Ball system_v13 (Autodesk Fusion 360 design; units mm, degrees)
Autodesk Fusion 360 part; units mm, degrees
sketch "Esquisse3" plane through (0, 0, 0) normal (1, 0, 0) x (0, 1, 0) in component "Ball unit"
  line L0 (0, 26) -> (0, 30)
  circle A0 centre (0, 20) radius 10
  line L1 (0, 0) -> (0, 20) construction
  line L2 (0, 0) -> (0, 10) construction
  line L3 (0, 20) -> (10, 20) construction
  line L4 (10, 20) -> (-10, 20)
  dimension "d8" = 4
  dimension "d9" = 20
  dimension "d10" = 20
  constraint vertical L0
  constraint coincident L0.end A0
  constraint coincident L1.start L2.start
  constraint coincident A0.centre L1.end
  constraint vertical L1
  constraint midpoint L1 L2.end
  constraint coincident A0 L3.end
  constraint perpendicular L1 L3
  constraint coincident A0 L4.end
  constraint perpendicular L1 L4
  measures "d8" distance of L0.start L0.end
  measures "d9" diameter of A0
  measures "d10" distance of L1.start A0.centre
sketch "Esquisse1" plane through (0, 0, 0) normal (0, 0, 1) x (1, 0, 0) in component "Ball unit"
  circle A0 centre (0, 0) radius 15
  circle A1 centre (0, 0) radius 4
  dimension "d1" = 30
  dimension "d2" = 8
  constraint coincident A0.centre A1.centre
  constraint concentric A0 A1
  measures "d1" diameter of A0
  measures "d2" diameter of A1
extrude "Extrusion1" add sketch "Esquisse1" along normal blind 26 contours A0 | A1 makes body 1 in component "Ball unit"
extrude "Extrusion2" add sketch "Esquisse1" against normal blind 25 contours A1 bodies 1 in component "Ball unit"
thread "Filetage1" "ISO Metric profile 8.0 M8x1.25 6g" major diameter 7.866 minor diameter 6.4455 pitch 1.25 angle 60 resizes the face on face at (3.9801, -0.3983, -8.3333) on bodies 1 in component "Ball unit"
sketch "Esquisse2" plane through (0, 0, 26) normal (0, 0, 1) x (-1, 0, 0) in component "Ball unit"
  circle A0 centre (0, 0) radius 15
  circle A1 centre (0, 0) radius 8.25
  dimension "d7" = 16.5
  constraint coincident A0.centre A1.centre
  measures "d7" diameter of A1
revolve "Révolution1" add sketch "Esquisse3" angle 360 about axis through (0, 10, 20) along (0, -1, 0) contours A0 L4 picked at (-0.0339, 23.8077) bodies 1 in component "Ball unit"
fillet "Congé1" radius 1 1 edges at (-13.9849, -5.4242, 26) on bodies 1 in component "Ball unit"
copy_body "CutPasteBodies1" bodies 1 removing the originals makes body 2 in component "Ball unit"
sketch "Esquisse1 (2)" plane through (0, 0, 0) normal (0, 0, 1) x (1, 0, 0) in component "Ball support"
  circle A0 centre (0, 0) radius 19
  circle A1 centre (0, 0) radius 4.5
  circle A2 centre (0, 0) radius 16
  circle A3 centre (0, 0) radius 7 construction
  line L0 (7, 4.0415) -> (0, 8.0829)
  line L1 (0, 8.0829) -> (-7, 4.0415)
  line L2 (-7, 4.0415) -> (-7, -4.0415)
  line L3 (-7, -4.0415) -> (0, -8.0829)
  line L4 (0, -8.0829) -> (7, -4.0415)
  line L5 (7, -4.0415) -> (7, 4.0415)
  dimension "d15" = 9
  dimension "d16" = 32
  dimension "d17" = 14
  dimension "d34" = 14
  dimension "d35" = 3
  constraint coincident A0.centre A1.centre
  constraint concentric A1 A2
  constraint concentric A1 A3
  constraint vertical L2
  measures "d15" diameter of A1
  measures "d16" diameter of A2
  measures "d17" diameter of A3
  measures "d34" distance of L1 L4
  measures "d35" distance of A0 A2
extrude "Extrusion1'" add sketch "Esquisse1 (2)" along normal blind 2 separate body contours A0 | A2 | L0 L1 L2 L3 L4 L5 makes body 3 in component "Ball support"
extrude "Extrusion2'" add sketch "Esquisse1 (2)" against normal blind 4 contours A0 | A2 bodies 3 in component "Ball support"
extrude "Extrusion3" add sketch "Esquisse1 (2)" against normal blind 20.7 contours A0 bodies 3 in component "Ball support"
sketch "Esquisse3 (2)" plane through (0, 0, -20.7) normal (0, 0, -1) x (1, 0, 0) in component "Ball support"
  circle A0 centre (0, 0) radius 16
  circle A1 centre (0, 0) radius 19
  line L0 (19, 0) -> (19, 4.7) construction
  circle A2 centre (0, 0) radius 19 construction
  line L1 (19, 4.7) -> (28.4, 4.7) construction
  line L2 (28.4, 4.7) -> (18.4095, 4.7)
  line L3 (18.4095, 4.7) -> (18.4095, -4.7) construction
  line L4 (18.4095, -4.7) -> (28.4, -4.7)
  line L5 (28.4, -4.7) -> (28.4, 4.7)
  line L6 (19, 0) -> (22, 0) construction
  circle A3 centre (23.7, 0) radius 1.7
  dimension "d37" = 4.7
  dimension "d39" = 9.4
  dimension "d40" = 9.4
  dimension "d41" = 3
  dimension "d42" = 3.4
  dimension "d43" = 4.7
  constraint vertical L0
  constraint tangent L0 A2
  constraint coincident L0.start A2
  constraint perpendicular L0 L1
  constraint horizontal L2
  constraint vertical L3
  constraint horizontal L4
  constraint vertical L5
  constraint coincident A2 L3.end
  constraint perpendicular L0 L6
  constraint coincident L6.end A3
  measures "d37" distance of L0.start L0.end
  measures "d39" distance of L0.end L1.end
  measures "d40" distance of L1.end L4.end
  measures "d41" distance of L0.start L6.end
  measures "d42" diameter of A3
  measures "d43" distance of L0.start A3.centre
extrude "Extrusion5" add sketch "Esquisse3 (2)" against normal blind 5 contours A1 L2 L4 L5 bodies 3 in component "Ball support"
fillet "Congé1'" radius 5 2 edges at (18.4095, 4.7, -18.2) (18.4095, -4.7, -18.2) on bodies 3 in component "Ball support"
chamfer "Chanfrein1" distance 1 angle 45 1 edges at (19, 0, -15.7) on bodies 3 in component "Ball support"
pattern_circular "Réseau C3" count 4 over 360 about axis through (0, 0, 1.75) along (0, 0, 1) of "Extrusion5", "Congé1'", "Chanfrein1" in component "Ball support"
sketch "Esquisse1 (3)" plane through (0, 0, 0) normal (0, 0, 1) x (1, 0, 0) in component "Nut"
  circle A0 centre (0, 0) radius 6.5 construction
  line L0 (6.5, 3.7528) -> (0, 7.5056)
  line L1 (0, 7.5056) -> (-6.5, 3.7528)
  line L2 (-6.5, 3.7528) -> (-6.5, -3.7528)
  line L3 (-6.5, -3.7528) -> (0, -7.5056)
  line L4 (0, -7.5056) -> (6.5, -3.7528)
  line L5 (6.5, -3.7528) -> (6.5, 3.7528)
  circle A1 centre (0, 0) radius 4
  dimension "d55" = 13
  dimension "d56" = 13
  dimension "d57" = 8
  constraint coincident A0.centre A1.centre
  constraint vertical L2
  constraint concentric A0 A1
  measures "d55" diameter of A0
  measures "d56" distance of L0 L3
  measures "d57" diameter of A1
extrude "Extrusion1''" add sketch "Esquisse1 (3)" against normal blind 6 separate body makes body 4 in component "Nut"
thread "Filetage1'" "ISO Metric profile 8.0 M8x1.25 6H" major diameter 8.17 minor diameter 6.7795 pitch 1.25 angle 60 resizes the face on face at (3.995, -0.1994, -4) on bodies 4 in component "Nut"
component "Ball unit" placed x (-1, 0, 0) y (0, 1, 0) z (0, 0, -1) at (0, 0, -9)
component "Ball support" placed x (1, 0, 0) y (0, 1, 0) z (0, 0, 1) at (0, 0, 0)
component "Nut" placed x (1, 0, 0) y (0, 1, 0) z (0, 0, 1) at (0, 0, 0)
component "Nut" placed x (1, 0, 0) y (0, 1, 0) z (0, 0, 1) at (0, 0, 8)
equation "d23 = -16.7 mm - 4 mm"
equation "d34 = d17"
equation "d35 = WallThickness"
equation "WallThickness = 3 mm"
equation "d37 = ( 3.4 / 2 ) * 1 mm + WallThickness"
equation "d39 = 3.4 mm + 2 * WallThickness"
equation "d40 = ( 4.7 * 2 ) * 1 mm"
equation "d56 = d55"
